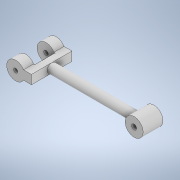
# Autodesk Inventor part: Tolerenced_Phalalnge_48mm
Saved by Autodesk Inventor 2021 (Build 250183000, 183)
## iProperties
Created: 2022-08-29
Part Number: Tolerenced_Phalalnge_48mm
Material: Generic
Document SubType Name: Modeling
Designer: alyn649
Density: 1 g/cm^3
Appearance: Default
Author: alyn649
Autodesk Inventor part; units mm, degrees
ref_plane "YZ Plane" through (0, 0, 0) normal (1, 0, 0) x (0, 1, 0)
ref_plane "XZ Plane" through (0, 0, 0) normal (0, 1, 0) x (-1, 0, 0)
ref_plane "XY Plane" through (0, 0, 0) normal (0, 0, 1) x (1, 0, 0)
sketch "Sketch1" plane through (0, 0, 0) normal (0, 0, 1) x (1, 0, 0)
  circle A0 centre (-24, 0) radius 1
  circle A1 centre (24, 0) radius 1
  circle A2 centre (-24, 0) radius 4
  circle A3 centre (24, 0) radius 4
  point P0 (0, 0)
  dimension "d0" = 2
  dimension "d1" = 2
  dimension "d3" = 48
  dimension "d4" = 24
  dimension "d5" = 8
  dimension "d6" = 8
  constraints: 4 centre point, 2 coincident, 2 horizontal alignment
  measures "d0" diameter of A0
  measures "d1" diameter of A1
  measures "d3" distance of A1.centre A0.centre
  measures "d4" distance of point (0, 0) A0.centre
  measures "d5" diameter of A2
  measures "d6" diameter of A3
extrude "Extrusion1" add sketch "Sketch1" against normal mid plane 18
sketch "Sketch2" plane through (0, 0, 0) normal (0, 0, 1) x (1, 0, 0)
  circle A0 centre (-24, 0) radius 4 projected
  circle A1 centre (-24, 0) radius 1 projected
  point P0 (0, 0)
extrude "Extrusion2" cut sketch "Sketch2" against normal mid plane 9
sketch "Sketch3" plane through (-24, 0, -4.5) normal (0, 0, 1) x (1, 0, 0)
  circle A0 centre (48, 0) radius 4 projected
  circle A1 centre (48, 0) radius 4 projected
  circle A2 centre (48, 0) radius 1 projected
  point P0 (24, 0)
extrude "Extrusion3" cut sketch "Sketch3" against normal blind 4.5
mirror "Mirror1" about plane through (0, 0, 0) normal (0, 0, 1) of "Extrusion3"
sketch "Sketch6" plane through (0, 0, 0) normal (0, 1, 0) x (-1, 0, 0)
  line L0 (-20, -4.5) -> (-23, -4.5) construction
  line L1 (-23, -4.5) -> (-23, 4.5) construction
  line L2 (-23, 4.5) -> (-20, 4.5) construction
  line L3 (-20, 4.5) -> (-20, -4.5) construction
  line L4 (-25, -4.5) -> (-28, -4.5) construction
  line L5 (-28, -4.5) -> (-28, 4.5) construction
  line L6 (-28, 4.5) -> (-25, 4.5) construction
  line L7 (-25, 4.5) -> (-25, -4.5) construction
  line L8 (20, 9) -> (23, 9) construction
  line L9 (23, 9) -> (23, 4.5) construction
  line L10 (23, 4.5) -> (20, 4.5) construction
  line L11 (20, 4.5) -> (20, 9) construction
  line L12 (25, 9) -> (28, 9) construction
  line L13 (28, 9) -> (28, 4.5) construction
  line L14 (28, 4.5) -> (25, 4.5) construction
  line L15 (25, 4.5) -> (25, 9) construction
  line L16 (28, -9) -> (25, -9) construction
  line L17 (25, -9) -> (25, -4.5) construction
  line L18 (25, -4.5) -> (28, -4.5) construction
  line L19 (28, -4.5) -> (28, -9) construction
  line L20 (23, -9) -> (20, -9) construction
  line L21 (20, -9) -> (20, -4.5) construction
  line L22 (20, -4.5) -> (23, -4.5) construction
  line L23 (23, -4.5) -> (23, -9) construction
  line L24 (20, -9) -> (28, -9) construction
  line L25 (20, -9) -> (17, -9)
  line L26 (17, -9) -> (17, -2)
  line L27 (17, -2) -> (-20, -2)
  line L28 (-20, 4.5) -> (-20, -4.5) construction
  line L29 (-20, 2) -> (17, 2)
  line L30 (17, 2) -> (17, 9)
  line L31 (17, 9) -> (20, 9)
  line L32 (20, -4.5) -> (28, -4.5) construction
  line L33 (20, -4.5) -> (20, 4.5)
  line L34 (-20, -2) -> (-23, -2)
  line L35 (-23, -4.5) -> (-23, 4.5) projected
  line L36 (-20, 2) -> (-23, 2)
  line L37 (20, -9) -> (23, -9)
  line L38 (23, -4.5) -> (20, -4.5)
  line L39 (25, -4.5) -> (23, -4.5) projected
  line L40 (23, -4.5) -> (23, -9)
  line L41 (23, -9) -> (23, -4.5) projected
  line L42 (23, 4.5) -> (25, 4.5) projected
  line L43 (28, 4.5) -> (20, 4.5) projected
  line L44 (23, 4.5) -> (20, 4.5)
  line L45 (23, 9) -> (25, 9) projected
  line L46 (23, 4.5) -> (23, 9)
  line L47 (28, 9) -> (20, 9) projected
  line L48 (23, 9) -> (20, 9)
  point P0 (0, 0)
  dimension "d16" = 3
  dimension "d17" = 4
  dimension "d18" = 2
  constraints: 30 end point, 6 perpendicular, 6 point on line, 3 collinear, 3 parallel, 1 horizontal, 1 vertical
  measures "d16" distance between parallel lines of L26 L21
  measures "d17" distance between parallel lines of L29 L27
  measures "d18" distance from line of point (0, 0) L27
extrude "Extrusion4" add sketch "Sketch6" against normal mid plane 4
sketch "Sketch7" plane through (-20, -2, -4.5) normal (-1, 0, 0) x (0, 0, 1)
  circle A0 centre (4.5, 2) radius 1
  dimension "d21" = 2
  constraints: 1 centre point, 1 coincident
  measures "d21" diameter of A0
extrude "Extrusion5" cut sketch "Sketch7" against normal blind 20
chamfer "Chamfer1" distance 1 angle 45 1 edges at (-20, 0, -1)
fillet "Fillet1" radius 2 4 edges at (1.7679, 2, 2) (1.7679, 2, -2) (1.7679, -2, -2) (1.7679, -2, 2)
sketch "Sketch9" plane through (0, 0, 9) normal (0, 0, 1) x (1, 0, 0)
  circle A0 centre (-24, 0) radius 1 projected
  circle A1 centre (-24, 0) radius 0.9
  point P0 (0, 0)
  dimension "d29" = 1.8
  constraints: 1 centre point, 1 coincident
  measures "d29" diameter of A1
extrude "TREAD" add sketch "Sketch9" against normal up to surface (4.5 mm away)
sketch "Sketch11" plane through (24, 0, 4.5) normal (0, 0, 1) x (1, 0, 0)
  circle A0 centre (0, 0) radius 4 projected
  circle A1 centre (0, 0) radius 1 projected
  point P0 (-24, 0)
extrude "thin" cut sketch "Sketch11" against normal blind 0.1
mirror "Mirror2" about plane through (0, 0, 0) normal (0, 0, 1) of "thin"
sketch "Sketch12" plane through (24, 0, 4.4) normal (0, 0, 1) x (1, 0, 0)
  circle A0 centre (0, 0) radius 1 construction
  circle A1 centre (0, 0) radius 1.1
  point P0 (-24, 0)
  dimension "d34" = 2.2
  constraints: 1 centre point, 1 coincident
  measures "d34" diameter of A1
extrude "Extrusion8" cut sketch "Sketch12" against normal up to surface (8.8 mm away)
equation "\"d4\" = 0.5 * d3"
equation "\"d6\" = d5"
equation "\"d18\" = 0.5 * d17"
body "Solid1"
